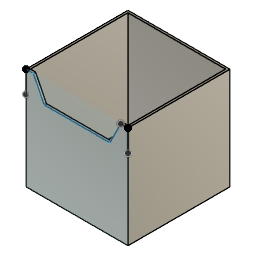
Storage_Box (Autodesk Fusion 360 design; units mm, degrees)
Autodesk Fusion 360 part; units mm, degrees
sketch "Sketch1" plane through (0, 0, 0) normal (0, 0, 1) x (1, 0, 0)
  line L0 (0, 0) -> (140, 0)
  line L1 (140, 0) -> (140, 140)
  line L2 (140, 140) -> (0, 140)
  line L3 (0, 140) -> (0, 0)
  dimension "d1" = 140
  dimension "d2" = 140
  constraint horizontal L0
  constraint vertical L1
  constraint horizontal L2
  constraint vertical L3
  constraint coincident L0.start L3.end
  measures "d1" distance of L0.start L0.end
  measures "d2" distance of L0.start L2.end
extrude "Extrude1" add sketch "Sketch1" along normal blind 140
sketch "Sketch2" plane through (0, 0, 140) normal (0, 0, 1) x (-1, 0, 0)
  line L0 (0, -140) -> (0, 0)
  line L1 (0, 0) -> (-140, 0)
  line L2 (-140, 0) -> (-140, -140)
  line L3 (-140, -140) -> (0, -140)
  line L4 (0, 0) -> (-3, 0)
  line L5 (-3, 0) -> (-3, -3)
  line L6 (-3, -3) -> (0, -3)
  line L7 (0, -3) -> (0, 0)
  line L8 (-140, -140) -> (-137, -140)
  line L9 (-137, -140) -> (-137, -137)
  line L10 (-137, -137) -> (-140, -137)
  line L11 (-140, -137) -> (-140, -140)
  line L12 (-3, -3) -> (-137, -3)
  line L13 (-137, -3) -> (-137, -137)
  line L14 (-137, -137) -> (-3, -137)
  line L15 (-3, -137) -> (-3, -3)
  dimension "d5" = 3
  dimension "d6" = 3
  dimension "d7" = 3
  dimension "d8" = 3
  constraint horizontal L4
  constraint vertical L5
  constraint horizontal L6
  constraint vertical L7
  constraint coincident L0.end L1.start
  constraint horizontal L8
  constraint vertical L9
  constraint horizontal L10
  constraint vertical L11
  constraint coincident L2.end L3.start
  constraint horizontal L12
  constraint vertical L13
  constraint horizontal L14
  constraint vertical L15
  measures "d5" distance of L0.end L4.end
  measures "d6" distance of L0.end L6.end
  measures "d7" distance of L2.end L8.end
  measures "d8" distance of L2.end L10.end
extrude "Extrude2" cut sketch "Sketch2" against normal blind 137 contours L12 L13 L14 L15
sketch "Sketch3" plane through (0, 0, 0) normal (0, -1, 0) x (1, 0, 0)
  line L0 (0, 0) -> (140, 0)
  line L1 (140, 0) -> (140, 140)
  line L2 (140, 140) -> (0, 140)
  line L3 (0, 140) -> (0, 0)
  line L4 (140, 110) -> (140, 140)
  line L5 (0, 140) -> (0, 110)
  line L6 (0, 140) -> (10, 140)
  line L7 (10, 140) -> (25, 110)
  line L8 (25, 110) -> (115, 110)
  line L9 (115, 110) -> (130, 140)
  line L10 (140, 140) -> (130, 140)
  constraint coincident L3 L5.end
  constraint coincident L1 L4.start
  constraint coincident L1.end L2.start
  constraint coincident L2.end L3.start
  constraint parallel L2 L8
  constraint coincident L2 L9.end
extrude "Extrude5" cut sketch "Sketch3" against normal blind 10 contours L2 L7 L8 L9
